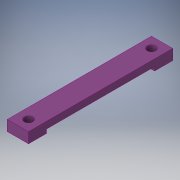
# Autodesk Inventor part: КВ33.044.305 - Прижим ремня
Saved by Autodesk Inventor 2019 (Build 230136000, 136)
## iProperties
Created: 2019-09-20
Part Number: КВ33.044.305 - Прижим ремня
Material: Пластик АБС
Document SubType Name: Modeling
Designer: Петров Иван
Density: 1.06 g/cm^3
Appearance: Гладкий — пурпурный
Author: Петров Иван
Autodesk Inventor part; units mm, degrees
ref_plane "YZ Plane" through (0, 0, 0) normal (1, 0, 0) x (0, 1, 0)
ref_plane "XZ Plane" through (0, 0, 0) normal (0, 1, 0) x (-1, 0, 0)
ref_plane "XY Plane" through (0, 0, 0) normal (0, 0, 1) x (1, 0, 0)
sketch "Эскиз1" plane through (0, 0, 0) normal (0, 1, 0) x (-1, 0, 0)
  line L0 (-8, -25.5) -> (-10, -25.5)
  line L1 (-10, -34) -> (-10, -25.5)
  line L2 (0, -34) -> (-10, -34)
  line L3 (0, -34) -> (0, -25.5)
  line L4 (0, -25.5) -> (-2, -25.5)
  line L5 (-2, -25.5) -> (-2, 25.5)
  line L6 (-2, 25.5) -> (0, 25.5)
  line L7 (0, 25.5) -> (0, 34)
  line L8 (0, 34) -> (-10, 34)
  line L9 (-10, 25.5) -> (-10, 34)
  line L10 (-10, 25.5) -> (-8, 25.5)
  line L11 (-8, 25.5) -> (-8, -25.5)
  line L12 (-4, 25.5) -> (-4, -25.5)
  line L13 (-4, -25.5) -> (-6, -25.5)
  line L14 (-6, -25.5) -> (-6, 25.5)
  line L15 (-6, 25.5) -> (-4, 25.5)
  circle A0 centre (-5, 29) radius 2
  circle A1 centre (-5, -29) radius 2
  line L16 (-10, 25.5) -> (-10, -25.5)
  line L17 (-10, -25.5) -> (-8, -25.5)
  line L18 (-8, -25.5) -> (-8, 25.5)
  line L19 (-8, 25.5) -> (-10, 25.5)
  line L20 (0, 25.5) -> (-2, 25.5)
  line L21 (-2, 25.5) -> (-2, -25.5)
  line L22 (-2, -25.5) -> (0, -25.5)
  line L23 (0, -25.5) -> (0, 25.5)
  point P0 (0, 0)
  point P1 (0, 0)
  constraints: 48 end point, 2 centre point
extrude "Выдавливание1" add sketch "Эскиз1" along normal blind 5 contours L11 L10 L9 L8 L7 L6 L5 L4 L3 L2 L1 L0 | L0 L16 L10 L11 | L4 L5 L6 L23 | L12 L13 L14 L15
sketch "Эскиз2" plane through (0, 0, 0) normal (0, -1, 0) x (1, 0, 0)
  line L0 (10, 34) -> (10, -34) projected
  line L1 (10, 0) -> (0, 0)
  line L2 (0, -34) -> (0, 34) projected
  line L3 (0, 25.5) -> (10, 25.5)
  line L4 (10, 25.5) -> (10, -25.5)
  line L5 (10, -25.5) -> (0, -25.5)
  line L6 (0, -25.5) -> (0, 25.5)
  line L7 (0, 25.5) -> (10, -25.5) construction
  line L8 (10, 25.5) -> (0, -25.5) construction
  point P0 (5, 0)
  dimension "d2" = 51
  constraints: 14 end point, 5 midpoint, 2 parallel, 1 horizontal, 1 perpendicular, 1 point on line
  measures "d2" distance of L3.end L4.end
extrude "Выдавливание2" cut sketch "Эскиз2" against normal blind 1.8
